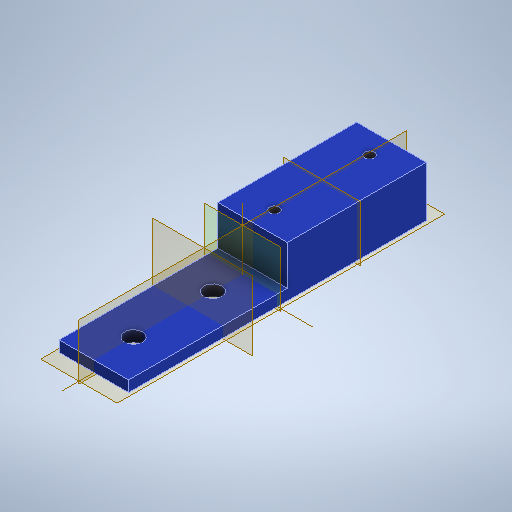
# Autodesk Inventor part: Adapterplatte_Vibrationsdaempfer
Saved by Autodesk Inventor 2025.2 (Build 292293000, 293)
## iProperties
Created: 2025-06-22
Part Number: Adapterplatte_Vibrationsdaempfer
Material: Generisch
Document SubType Name: Modeling
Designer: Jakob
Density: 1 g/cm^3
Appearance: Vorgabe
Author: Jakob
Autodesk Inventor part; units mm, degrees
sketch "Skizze1" plane through (0, 0, 0) normal (0, 0, 1) x (1, 0, 0)
  line L0 (-17.5, 75) -> (17.5, 75)
  line L1 (17.5, 75) -> (17.5, -75)
  line L2 (17.5, -75) -> (-17.5, -75)
  line L3 (-17.5, -75) -> (-17.5, 75)
  line L4 (-17.5, 75) -> (17.5, -75) construction
  line L5 (17.5, 75) -> (-17.5, -75) construction
  point P0 (0, 0)
  dimension "d0" = 35
  dimension "d1" = 150
  constraints: 12 end point, 2 midpoint, 2 parallel, 1 horizontal, 1 perpendicular
  measures "d0" distance of L0.start L0.end
  measures "d1" distance of L0.end L1.end
extrude "Extrusion1" add sketch "Skizze1" along normal blind 5.5
sketch "Skizze3" plane through (0, 0, 5.5) normal (0, 0, 1) x (1, 0, 0)
  line L0 (-17.5, 5) -> (17.5, 5)
  line L1 (17.5, 5) -> (17.5, 75)
  line L2 (17.5, 75) -> (-17.5, 75)
  line L3 (-17.5, 75) -> (-17.5, 5)
  line L4 (-17.5, 5) -> (17.5, 75) construction
  line L5 (17.5, 5) -> (-17.5, 75) construction
  line L6 (-17.5, 75) -> (-17.5, -75) projected
  line L7 (17.5, 75) -> (-17.5, 75) projected
  line L8 (17.5, -75) -> (17.5, 75) projected
  point P0 (0, 40)
  point P1 (-4.35, 75)
  point P2 (-17.5, 40)
  dimension "d8" = 70
  constraints: 12 end point, 3 collinear, 3 midpoint, 2 parallel, 1 horizontal, 1 perpendicular
  measures "d8" distance of L2.end L0.start
extrude "Extrusion3" add sketch "Skizze3" along normal blind 20
ref_plane "Arbeitsebene2" through (-17.5, 40, 5.5) normal (0, -1, 0) x (1, 0, 0)
sketch "Skizze5" plane through (0, 0, 25.5) normal (0, 0, 1) x (1, 0, 0)
  line L0 (24.5, 40) -> (-24.5, 40) projected
  line L1 (0, 105) -> (0, -105) projected
  point P0 (0, 0)
  point P1 (0, 16)
  point P2 (0, 64)
  dimension "d23" = 24
  dimension "d24" = 24
  constraints: 2 point on line
  measures "d23" distance from line of L0 point (0, 16)
  measures "d24" distance from line of L0 point (0, 64)
hole "Bohrung2" at (0, 16, 25.5) at (0, 64, 25.5) direction (0, 0, -1) diameter 4.917 depth 16 tip angle 118 thread size "M6x1" class "6H" standard "ISO Metric profile"
ref_plane "Arbeitsebene3" through (-17.5, -27.5, 0) normal (0, -1, 0) x (1, 0, 0)
sketch "Skizze6" plane through (0, 0, 5.5) normal (0, 0, 1) x (1, 0, 0)
  line L0 (0, 105) -> (0, -105) projected
  line L1 (-17.5, -75) -> (17.5, -75) projected
  point P0 (0, 0)
  point P1 (0, -55)
  point P2 (0, -15)
  dimension "d36" = 20
  dimension "d37" = 60
  constraints: 2 point on line
  measures "d36" distance from line of L1 point (0, -55)
  measures "d37" distance from line of L1 point (0, -15)
hole "Bohrung3" at (0, -55, 5.5) at (0, -15, 5.5) direction (0, 0, -1) diameter 9 end through all clearance for "Flachkopfsenkschraube DIN EN ISO 2009" size "M8" standard "DIN"
